Autodesk Fusion 360 part; units mm, degrees
(part 3 of 3)
sketch "Schizzo3" plane through (0, 0, 22) normal (0, 0, 1) x (-1, 0, 0)
  line L0 (-2.6533, 1.4) -> (2.6533, 1.4)
  arc A0 (-2.6533, 1.4) -> (2.6533, 1.4) centre (0, 0) ccw
  circle A1 centre (0, 0) radius 30.1547
  circle A2 centre (0, 30.1547) radius 0.5
  dimension "d10" = 1
  constraint coincident A1 A2.centre
  measures "d10" diameter of A2
extrude "Estrusione4" cut sketch "Schizzo3" against normal through all contours A1 A2 picked at (0.0124, 29.9882)
pattern_circular "Serie C1" count 120 over 360 about axis through (0, 0, 2) along (0, 0, 1) of "Estrusione4"
sketch "Schizzo4" plane through (0, 0, 22) normal (0, 0, 1) x (-1, 0, 0)
  arc A0 (1.0787, 30.1354) -> (2.0773, 30.0831) centre (1.5782, 30.1134) ccw
  arc A1 (1.0787, 30.1354) -> (0.5, 30.1506) centre (0, 0) ccw
  arc A2 (-0.5, 30.1506) -> (0.5, 30.1506) centre (0, 30.1547) ccw
  arc A3 (-0.5, 30.1506) -> (-1.0787, 30.1354) centre (0, 0) ccw
  arc A4 (-2.0773, 30.0831) -> (-1.0787, 30.1354) centre (-1.5782, 30.1134) ccw
  arc A5 (-2.0773, 30.0831) -> (-2.6543, 30.0376) centre (0, 0) ccw
  arc A6 (-3.6488, 29.9331) -> (-2.6543, 30.0376) centre (-3.152, 29.9895) ccw
  arc A7 (-3.6488, 29.9331) -> (-4.2228, 29.8576) centre (0, 0) ccw
  arc A8 (-5.2104, 29.7011) -> (-4.2228, 29.8576) centre (-4.7172, 29.7834) ccw
  arc A9 (-5.2104, 29.7011) -> (-5.7796, 29.5956) centre (0, 0) ccw
  arc A10 (-6.7577, 29.3877) -> (-5.7796, 29.5956) centre (-6.2695, 29.4957) ccw
  arc A11 (-6.7577, 29.3877) -> (-7.3206, 29.2526) centre (0, 0) ccw
  arc A12 (-8.2865, 28.9938) -> (-7.3206, 29.2526) centre (-7.8046, 29.1272) ccw
  arc A13 (-8.2865, 28.9938) -> (-8.8415, 28.8294) centre (0, 0) ccw
  arc A14 (-9.7925, 28.5204) -> (-8.8415, 28.8294) centre (-9.3183, 28.6788) ccw
  arc A15 (-9.7925, 28.5204) -> (-10.3382, 28.3271) centre (0, 0) ccw
  arc A16 (-11.2718, 27.9688) -> (-10.3382, 28.3271) centre (-10.8065, 28.1518) ccw
  arc A17 (-11.2718, 27.9688) -> (-11.8066, 27.7473) centre (0, 0) ccw
  arc A18 (-12.7201, 27.3405) -> (-11.8066, 27.7473) centre (-12.265, 27.5477) ccw
  arc A19 (-12.7201, 27.3405) -> (-13.2426, 27.0913) centre (0, 0) ccw
  arc A20 (-14.1336, 26.6374) -> (-13.2426, 27.0913) centre (-13.6899, 26.868) ccw
  arc A21 (-14.1336, 26.6374) -> (-14.6423, 26.3611) centre (0, 0) ccw
  arc A22 (-15.5083, 25.8612) -> (-14.6423, 26.3611) centre (-15.0774, 26.1147) ccw
  arc A23 (-15.5083, 25.8612) -> (-16.0018, 25.5587) centre (0, 0) ccw
  arc A24 (-16.8405, 25.0141) -> (-16.0018, 25.5587) centre (-16.4234, 25.2899) ccw
  arc A25 (-16.8405, 25.0141) -> (-17.3176, 24.6862) centre (0, 0) ccw
  arc A26 (-18.1265, 24.0984) -> (-17.3176, 24.6862) centre (-17.7245, 24.3957) ccw
  arc A27 (-18.1265, 24.0984) -> (-18.5858, 23.746) centre (0, 0) ccw
  arc A28 (-19.3629, 23.1167) -> (-18.5858, 23.746) centre (-18.977, 23.4346) ccw
  arc A29 (-19.3629, 23.1167) -> (-19.8031, 22.7408) centre (0, 0) ccw
  arc A30 (-20.5462, 22.0717) -> (-19.8031, 22.7408) centre (-20.1774, 22.4093) ccw
  arc A31 (-20.5462, 22.0717) -> (-20.9661, 21.6732) centre (0, 0) ccw
  arc A32 (-21.6732, 20.9661) -> (-20.9661, 21.6732) centre (-21.3226, 21.3226) ccw
  arc A33 (-21.6732, 20.9661) -> (-22.0717, 20.5462) centre (0, 0) ccw
  arc A34 (-22.7408, 19.8031) -> (-22.0717, 20.5462) centre (-22.4093, 20.1774) ccw
  arc A35 (-22.7408, 19.8031) -> (-23.1167, 19.3629) centre (0, 0) ccw
  arc A36 (-23.746, 18.5858) -> (-23.1167, 19.3629) centre (-23.4346, 18.977) ccw
  arc A37 (-23.746, 18.5858) -> (-24.0984, 18.1265) centre (0, 0) ccw
  arc A38 (-24.6862, 17.3176) -> (-24.0984, 18.1265) centre (-24.3957, 17.7245) ccw
  arc A39 (-24.6862, 17.3176) -> (-25.0141, 16.8405) centre (0, 0) ccw
  arc A40 (-25.5587, 16.0018) -> (-25.0141, 16.8405) centre (-25.2899, 16.4234) ccw
  arc A41 (-25.5587, 16.0018) -> (-25.8612, 15.5083) centre (0, 0) ccw
  arc A42 (-26.3611, 14.6423) -> (-25.8612, 15.5083) centre (-26.1147, 15.0774) ccw
  arc A43 (-26.3611, 14.6423) -> (-26.6374, 14.1336) centre (0, 0) ccw
  arc A44 (-27.0913, 13.2426) -> (-26.6374, 14.1336) centre (-26.868, 13.6899) ccw
  arc A45 (-27.0913, 13.2426) -> (-27.3405, 12.7201) centre (0, 0) ccw
  arc A46 (-27.7473, 11.8066) -> (-27.3405, 12.7201) centre (-27.5477, 12.265) ccw
  arc A47 (-27.7473, 11.8066) -> (-27.9688, 11.2718) centre (0, 0) ccw
  arc A48 (-28.3271, 10.3382) -> (-27.9688, 11.2718) centre (-28.1518, 10.8065) ccw
  arc A49 (-28.3271, 10.3382) -> (-28.5204, 9.7925) centre (0, 0) ccw
  arc A50 (-28.8294, 8.8415) -> (-28.5204, 9.7925) centre (-28.6788, 9.3183) ccw
  arc A51 (-28.8294, 8.8415) -> (-28.9938, 8.2865) centre (0, 0) ccw
  arc A52 (-29.2526, 7.3206) -> (-28.9938, 8.2865) centre (-29.1272, 7.8046) ccw
  arc A53 (-29.2526, 7.3206) -> (-29.3877, 6.7577) centre (0, 0) ccw
  arc A54 (-29.5956, 5.7796) -> (-29.3877, 6.7577) centre (-29.4957, 6.2695) ccw
  arc A55 (-29.5956, 5.7796) -> (-29.7011, 5.2104) centre (0, 0) ccw
  arc A56 (-29.8576, 4.2228) -> (-29.7011, 5.2104) centre (-29.7834, 4.7172) ccw
  arc A57 (-29.8576, 4.2228) -> (-29.9331, 3.6488) centre (0, 0) ccw
  arc A58 (-30.0376, 2.6543) -> (-29.9331, 3.6488) centre (-29.9895, 3.152) ccw
  arc A59 (-30.0376, 2.6543) -> (-30.0831, 2.0773) centre (0, 0) ccw
  arc A60 (-30.1354, 1.0787) -> (-30.0831, 2.0773) centre (-30.1134, 1.5782) ccw
  arc A61 (-30.1354, 1.0787) -> (-30.1506, 0.5) centre (0, 0) ccw
  arc A62 (-30.1506, -0.5) -> (-30.1506, 0.5) centre (-30.1547, 0) ccw
  arc A63 (-30.1506, -0.5) -> (-30.1354, -1.0787) centre (0, 0) ccw
  arc A64 (-30.0831, -2.0773) -> (-30.1354, -1.0787) centre (-30.1134, -1.5782) ccw
  arc A65 (-30.0831, -2.0773) -> (-30.0376, -2.6543) centre (0, 0) ccw
  arc A66 (-29.9331, -3.6488) -> (-30.0376, -2.6543) centre (-29.9895, -3.152) ccw
  arc A67 (-29.9331, -3.6488) -> (-29.8576, -4.2228) centre (0, 0) ccw
  arc A68 (-29.7011, -5.2104) -> (-29.8576, -4.2228) centre (-29.7834, -4.7172) ccw
  arc A69 (-29.7011, -5.2104) -> (-29.5956, -5.7796) centre (0, 0) ccw
  arc A70 (-29.3877, -6.7577) -> (-29.5956, -5.7796) centre (-29.4957, -6.2695) ccw
  arc A71 (-29.3877, -6.7577) -> (-29.2526, -7.3206) centre (0, 0) ccw
  arc A72 (-28.9938, -8.2865) -> (-29.2526, -7.3206) centre (-29.1272, -7.8046) ccw
  arc A73 (-28.9938, -8.2865) -> (-28.8294, -8.8415) centre (0, 0) ccw
  arc A74 (-28.5204, -9.7925) -> (-28.8294, -8.8415) centre (-28.6788, -9.3183) ccw
  arc A75 (-28.5204, -9.7925) -> (-28.3271, -10.3382) centre (0, 0) ccw
  arc A76 (-27.9688, -11.2718) -> (-28.3271, -10.3382) centre (-28.1518, -10.8065) ccw
  arc A77 (-27.9688, -11.2718) -> (-27.7473, -11.8066) centre (0, 0) ccw
  arc A78 (-27.3405, -12.7201) -> (-27.7473, -11.8066) centre (-27.5477, -12.265) ccw
  arc A79 (-27.3405, -12.7201) -> (-27.0913, -13.2426) centre (0, 0) ccw
  arc A80 (-26.6374, -14.1336) -> (-27.0913, -13.2426) centre (-26.868, -13.6899) ccw
  arc A81 (-26.6374, -14.1336) -> (-26.3611, -14.6423) centre (0, 0) ccw
  arc A82 (-25.8612, -15.5083) -> (-26.3611, -14.6423) centre (-26.1147, -15.0774) ccw
  arc A83 (-25.8612, -15.5083) -> (-25.5587, -16.0018) centre (0, 0) ccw
  arc A84 (-25.0141, -16.8405) -> (-25.5587, -16.0018) centre (-25.2899, -16.4234) ccw
  arc A85 (-25.0141, -16.8405) -> (-24.6862, -17.3176) centre (0, 0) ccw
  arc A86 (-24.0984, -18.1265) -> (-24.6862, -17.3176) centre (-24.3957, -17.7245) ccw
  arc A87 (-24.0984, -18.1265) -> (-23.746, -18.5858) centre (0, 0) ccw
  arc A88 (-23.1167, -19.3629) -> (-23.746, -18.5858) centre (-23.4346, -18.977) ccw
  arc A89 (-23.1167, -19.3629) -> (-22.7408, -19.8031) centre (0, 0) ccw
  arc A90 (-22.0717, -20.5462) -> (-22.7408, -19.8031) centre (-22.4093, -20.1774) ccw
  arc A91 (-22.0717, -20.5462) -> (-21.6732, -20.9661) centre (0, 0) ccw
  arc A92 (-20.9661, -21.6732) -> (-21.6732, -20.9661) centre (-21.3226, -21.3226) ccw
  arc A93 (-20.9661, -21.6732) -> (-20.5462, -22.0717) centre (0, 0) ccw
  arc A94 (-19.8031, -22.7408) -> (-20.5462, -22.0717) centre (-20.1774, -22.4093) ccw
  arc A95 (-19.8031, -22.7408) -> (-19.3629, -23.1167) centre (0, 0) ccw
  arc A96 (-18.5858, -23.746) -> (-19.3629, -23.1167) centre (-18.977, -23.4346) ccw
  arc A97 (-18.5858, -23.746) -> (-18.1265, -24.0984) centre (0, 0) ccw
  arc A98 (-17.3176, -24.6862) -> (-18.1265, -24.0984) centre (-17.7245, -24.3957) ccw
  arc A99 (-17.3176, -24.6862) -> (-16.8405, -25.0141) centre (0, 0) ccw
  arc A100 (-16.0018, -25.5587) -> (-16.8405, -25.0141) centre (-16.4234, -25.2899) ccw
  arc A101 (-16.0018, -25.5587) -> (-15.5083, -25.8612) centre (0, 0) ccw
  arc A102 (-14.6423, -26.3611) -> (-15.5083, -25.8612) centre (-15.0774, -26.1147) ccw
  arc A103 (-14.6423, -26.3611) -> (-14.1336, -26.6374) centre (0, 0) ccw
  arc A104 (-13.2426, -27.0913) -> (-14.1336, -26.6374) centre (-13.6899, -26.868) ccw
  arc A105 (-13.2426, -27.0913) -> (-12.7201, -27.3405) centre (0, 0) ccw
  arc A106 (-11.8066, -27.7473) -> (-12.7201, -27.3405) centre (-12.265, -27.5477) ccw
  arc A107 (-11.8066, -27.7473) -> (-11.2718, -27.9688) centre (0, 0) ccw
  arc A108 (-10.3382, -28.3271) -> (-11.2718, -27.9688) centre (-10.8065, -28.1518) ccw
  arc A109 (-10.3382, -28.3271) -> (-9.7925, -28.5204) centre (0, 0) ccw
  arc A110 (-8.8415, -28.8294) -> (-9.7925, -28.5204) centre (-9.3183, -28.6788) ccw
  arc A111 (-8.8415, -28.8294) -> (-8.2865, -28.9938) centre (0, 0) ccw
  arc A112 (-7.3206, -29.2526) -> (-8.2865, -28.9938) centre (-7.8046, -29.1272) ccw
  arc A113 (-7.3206, -29.2526) -> (-6.7577, -29.3877) centre (0, 0) ccw
  arc A114 (-5.7796, -29.5956) -> (-6.7577, -29.3877) centre (-6.2695, -29.4957) ccw
  arc A115 (-5.7796, -29.5956) -> (-5.2104, -29.7011) centre (0, 0) ccw
  arc A116 (-4.2228, -29.8576) -> (-5.2104, -29.7011) centre (-4.7172, -29.7834) ccw
  arc A117 (-4.2228, -29.8576) -> (-3.6488, -29.9331) centre (0, 0) ccw
  arc A118 (-2.6543, -30.0376) -> (-3.6488, -29.9331) centre (-3.152, -29.9895) ccw
  arc A119 (-2.6543, -30.0376) -> (-2.0773, -30.0831) centre (0, 0) ccw
  arc A120 (-1.0787, -30.1354) -> (-2.0773, -30.0831) centre (-1.5782, -30.1134) ccw
  arc A121 (-1.0787, -30.1354) -> (-0.5, -30.1506) centre (0, 0) ccw
  arc A122 (0.5, -30.1506) -> (-0.5, -30.1506) centre (0, -30.1547) ccw
  arc A123 (0.5, -30.1506) -> (1.0787, -30.1354) centre (0, 0) ccw
  arc A124 (2.0773, -30.0831) -> (1.0787, -30.1354) centre (1.5782, -30.1134) ccw
  arc A125 (2.0773, -30.0831) -> (2.6543, -30.0376) centre (0, 0) ccw
  arc A126 (3.6488, -29.9331) -> (2.6543, -30.0376) centre (3.152, -29.9895) ccw
  arc A127 (3.6488, -29.9331) -> (4.2228, -29.8576) centre (0, 0) ccw
  arc A128 (5.2104, -29.7011) -> (4.2228, -29.8576) centre (4.7172, -29.7834) ccw
  arc A129 (5.2104, -29.7011) -> (5.7796, -29.5956) centre (0, 0) ccw
  arc A130 (6.7577, -29.3877) -> (5.7796, -29.5956) centre (6.2695, -29.4957) ccw
  arc A131 (6.7577, -29.3877) -> (7.3206, -29.2526) centre (0, 0) ccw
  arc A132 (8.2865, -28.9938) -> (7.3206, -29.2526) centre (7.8046, -29.1272) ccw
  arc A133 (8.2865, -28.9938) -> (8.8415, -28.8294) centre (0, 0) ccw
  arc A134 (9.7925, -28.5204) -> (8.8415, -28.8294) centre (9.3183, -28.6788) ccw
  arc A135 (9.7925, -28.5204) -> (10.3382, -28.3271) centre (0, 0) ccw
  arc A136 (11.2718, -27.9688) -> (10.3382, -28.3271) centre (10.8065, -28.1518) ccw
  arc A137 (11.2718, -27.9688) -> (11.8066, -27.7473) centre (0, 0) ccw
  arc A138 (12.7201, -27.3405) -> (11.8066, -27.7473) centre (12.265, -27.5477) ccw
  arc A139 (12.7201, -27.3405) -> (13.2426, -27.0913) centre (0, 0) ccw
  arc A140 (14.1336, -26.6374) -> (13.2426, -27.0913) centre (13.6899, -26.868) ccw
  arc A141 (14.1336, -26.6374) -> (14.6423, -26.3611) centre (0, 0) ccw
  arc A142 (15.5083, -25.8612) -> (14.6423, -26.3611) centre (15.0774, -26.1147) ccw
  arc A143 (15.5083, -25.8612) -> (16.0018, -25.5587) centre (0, 0) ccw
  arc A144 (16.8405, -25.0141) -> (16.0018, -25.5587) centre (16.4234, -25.2899) ccw
  arc A145 (16.8405, -25.0141) -> (17.3176, -24.6862) centre (0, 0) ccw
  arc A146 (18.1265, -24.0984) -> (17.3176, -24.6862) centre (17.7245, -24.3957) ccw
  arc A147 (18.1265, -24.0984) -> (18.5858, -23.746) centre (0, 0) ccw
  arc A148 (19.3629, -23.1167) -> (18.5858, -23.746) centre (18.977, -23.4346) ccw
  arc A149 (19.3629, -23.1167) -> (19.8031, -22.7408) centre (0, 0) ccw
  arc A150 (20.5462, -22.0717) -> (19.8031, -22.7408) centre (20.1774, -22.4093) ccw
  arc A151 (20.5462, -22.0717) -> (20.9661, -21.6732) centre (0, 0) ccw
  arc A152 (21.6732, -20.9661) -> (20.9661, -21.6732) centre (21.3226, -21.3226) ccw
  arc A153 (21.6732, -20.9661) -> (22.0717, -20.5462) centre (0, 0) ccw
  arc A154 (22.7408, -19.8031) -> (22.0717, -20.5462) centre (22.4093, -20.1774) ccw
  arc A155 (22.7408, -19.8031) -> (23.1167, -19.3629) centre (0, 0) ccw
  arc A156 (23.746, -18.5858) -> (23.1167, -19.3629) centre (23.4346, -18.977) ccw
  arc A157 (23.746, -18.5858) -> (24.0984, -18.1265) centre (0, 0) ccw
  arc A158 (24.6862, -17.3176) -> (24.0984, -18.1265) centre (24.3957, -17.7245) ccw
  arc A159 (24.6862, -17.3176) -> (25.0141, -16.8405) centre (0, 0) ccw
  arc A160 (25.5587, -16.0018) -> (25.0141, -16.8405) centre (25.2899, -16.4234) ccw
  arc A161 (25.5587, -16.0018) -> (25.8612, -15.5083) centre (0, 0) ccw
  arc A162 (26.3611, -14.6423) -> (25.8612, -15.5083) centre (26.1147, -15.0774) ccw
  arc A163 (26.3611, -14.6423) -> (26.6374, -14.1336) centre (0, 0) ccw
  arc A164 (27.0913, -13.2426) -> (26.6374, -14.1336) centre (26.868, -13.6899) ccw
  arc A165 (27.0913, -13.2426) -> (27.3405, -12.7201) centre (0, 0) ccw
  arc A166 (27.7473, -11.8066) -> (27.3405, -12.7201) centre (27.5477, -12.265) ccw
  arc A167 (27.7473, -11.8066) -> (27.9688, -11.2718) centre (0, 0) ccw
  arc A168 (28.3271, -10.3382) -> (27.9688, -11.2718) centre (28.1518, -10.8065) ccw
  arc A169 (28.3271, -10.3382) -> (28.5204, -9.7925) centre (0, 0) ccw
  arc A170 (28.8294, -8.8415) -> (28.5204, -9.7925) centre (28.6788, -9.3183) ccw
  arc A171 (28.8294, -8.8415) -> (28.9938, -8.2865) centre (0, 0) ccw
  arc A172 (29.2526, -7.3206) -> (28.9938, -8.2865) centre (29.1272, -7.8046) ccw
  arc A173 (29.2526, -7.3206) -> (29.3877, -6.7577) centre (0, 0) ccw
  arc A174 (29.5956, -5.7796) -> (29.3877, -6.7577) centre (29.4957, -6.2695) ccw
  arc A175 (29.5956, -5.7796) -> (29.7011, -5.2104) centre (0, 0) ccw
  arc A176 (29.8576, -4.2228) -> (29.7011, -5.2104) centre (29.7834, -4.7172) ccw
  arc A177 (29.8576, -4.2228) -> (29.9331, -3.6488) centre (0, 0) ccw
  arc A178 (30.0376, -2.6543) -> (29.9331, -3.6488) centre (29.9895, -3.152) ccw
  arc A179 (30.0376, -2.6543) -> (30.0831, -2.0773) centre (0, 0) ccw
  arc A180 (30.1354, -1.0787) -> (30.0831, -2.0773) centre (30.1134, -1.5782) ccw
  arc A181 (30.1354, -1.0787) -> (30.1506, -0.5) centre (0, 0) ccw
  arc A182 (30.1506, 0.5) -> (30.1506, -0.5) centre (30.1547, 0) ccw
  arc A183 (30.1506, 0.5) -> (30.1354, 1.0787) centre (0, 0) ccw
  arc A184 (30.0831, 2.0773) -> (30.1354, 1.0787) centre (30.1134, 1.5782) ccw
  arc A185 (30.0831, 2.0773) -> (30.0376, 2.6543) centre (0, 0) ccw
  arc A186 (29.9331, 3.6488) -> (30.0376, 2.6543) centre (29.9895, 3.152) ccw
  arc A187 (29.9331, 3.6488) -> (29.8576, 4.2228) centre (0, 0) ccw
  arc A188 (29.7011, 5.2104) -> (29.8576, 4.2228) centre (29.7834, 4.7172) ccw
  arc A189 (29.7011, 5.2104) -> (29.5956, 5.7796) centre (0, 0) ccw
  arc A190 (29.3877, 6.7577) -> (29.5956, 5.7796) centre (29.4957, 6.2695) ccw
  arc A191 (29.3877, 6.7577) -> (29.2526, 7.3206) centre (0, 0) ccw
  arc A192 (28.9938, 8.2865) -> (29.2526, 7.3206) centre (29.1272, 7.8046) ccw
  arc A193 (28.9938, 8.2865) -> (28.8294, 8.8415) centre (0, 0) ccw
  arc A194 (28.5204, 9.7925) -> (28.8294, 8.8415) centre (28.6788, 9.3183) ccw
  arc A195 (28.5204, 9.7925) -> (28.3271, 10.3382) centre (0, 0) ccw
  arc A196 (27.9688, 11.2718) -> (28.3271, 10.3382) centre (28.1518, 10.8065) ccw
  arc A197 (27.9688, 11.2718) -> (27.7473, 11.8066) centre (0, 0) ccw
  arc A198 (27.3405, 12.7201) -> (27.7473, 11.8066) centre (27.5477, 12.265) ccw
  arc A199 (27.3405, 12.7201) -> (27.0913, 13.2426) centre (0, 0) ccw
  arc A200 (26.6374, 14.1336) -> (27.0913, 13.2426) centre (26.868, 13.6899) ccw
  arc A201 (26.6374, 14.1336) -> (26.3611, 14.6423) centre (0, 0) ccw
  arc A202 (25.8612, 15.5083) -> (26.3611, 14.6423) centre (26.1147, 15.0774) ccw
  arc A203 (25.8612, 15.5083) -> (25.5587, 16.0018) centre (0, 0) ccw
  arc A204 (25.0141, 16.8405) -> (25.5587, 16.0018) centre (25.2899, 16.4234) ccw
  arc A205 (25.0141, 16.8405) -> (24.6862, 17.3176) centre (0, 0) ccw
  arc A206 (24.0984, 18.1265) -> (24.6862, 17.3176) centre (24.3957, 17.7245) ccw
  arc A207 (24.0984, 18.1265) -> (23.746, 18.5858) centre (0, 0) ccw
  arc A208 (23.1167, 19.3629) -> (23.746, 18.5858) centre (23.4346, 18.977) ccw
  arc A209 (23.1167, 19.3629) -> (22.7408, 19.8031) centre (0, 0) ccw
  arc A210 (22.0717, 20.5462) -> (22.7408, 19.8031) centre (22.4093, 20.1774) ccw
  arc A211 (22.0717, 20.5462) -> (21.6732, 20.9661) centre (0, 0) ccw
  arc A212 (20.9661, 21.6732) -> (21.6732, 20.9661) centre (21.3226, 21.3226) ccw
  arc A213 (20.9661, 21.6732) -> (20.5462, 22.0717) centre (0, 0) ccw
  arc A214 (19.8031, 22.7408) -> (20.5462, 22.0717) centre (20.1774, 22.4093) ccw
  arc A215 (19.8031, 22.7408) -> (19.3629, 23.1167) centre (0, 0) ccw
  arc A216 (18.5858, 23.746) -> (19.3629, 23.1167) centre (18.977, 23.4346) ccw
  arc A217 (18.5858, 23.746) -> (18.1265, 24.0984) centre (0, 0) ccw
  arc A218 (17.3176, 24.6862) -> (18.1265, 24.0984) centre (17.7245, 24.3957) ccw
  arc A219 (17.3176, 24.6862) -> (16.8405, 25.0141) centre (0, 0) ccw
  arc A220 (16.0018, 25.5587) -> (16.8405, 25.0141) centre (16.4234, 25.2899) ccw
  arc A221 (16.0018, 25.5587) -> (15.5083, 25.8612) centre (0, 0) ccw
  arc A222 (14.6423, 26.3611) -> (15.5083, 25.8612) centre (15.0774, 26.1147) ccw
  arc A223 (14.6423, 26.3611) -> (14.1336, 26.6374) centre (0, 0) ccw
  arc A224 (13.2426, 27.0913) -> (14.1336, 26.6374) centre (13.6899, 26.868) ccw
  arc A225 (13.2426, 27.0913) -> (12.7201, 27.3405) centre (0, 0) ccw
  arc A226 (11.8066, 27.7473) -> (12.7201, 27.3405) centre (12.265, 27.5477) ccw
  arc A227 (11.8066, 27.7473) -> (11.2718, 27.9688) centre (0, 0) ccw
  arc A228 (10.3382, 28.3271) -> (11.2718, 27.9688) centre (10.8065, 28.1518) ccw
  arc A229 (10.3382, 28.3271) -> (9.7925, 28.5204) centre (0, 0) ccw
  arc A230 (8.8415, 28.8294) -> (9.7925, 28.5204) centre (9.3183, 28.6788) ccw
  arc A231 (8.8415, 28.8294) -> (8.2865, 28.9938) centre (0, 0) ccw
  arc A232 (7.3206, 29.2526) -> (8.2865, 28.9938) centre (7.8046, 29.1272) ccw
  arc A233 (7.3206, 29.2526) -> (6.7577, 29.3877) centre (0, 0) ccw
  arc A234 (5.7796, 29.5956) -> (6.7577, 29.3877) centre (6.2695, 29.4957) ccw
  arc A235 (5.7796, 29.5956) -> (5.2104, 29.7011) centre (0, 0) ccw
  arc A236 (4.2228, 29.8576) -> (5.2104, 29.7011) centre (4.7172, 29.7834) ccw
  arc A237 (4.2228, 29.8576) -> (3.6488, 29.9331) centre (0, 0) ccw
  arc A238 (2.6543, 30.0376) -> (3.6488, 29.9331) centre (3.152, 29.9895) ccw
  arc A239 (2.6543, 30.0376) -> (2.0773, 30.0831) centre (0, 0) ccw
  line L0 (-2.6533, 1.4) -> (2.6533, 1.4)
  arc A240 (-2.6533, 1.4) -> (2.6533, 1.4) centre (0, 0) ccw
  circle A241 centre (0, 0) radius 26.2291
  circle A242 centre (0, 0) radius 7.0711
  constraint coincident A1.centre A3.centre
extrude "Estrusione5" cut sketch "Schizzo4" against normal blind 18 contours A241
